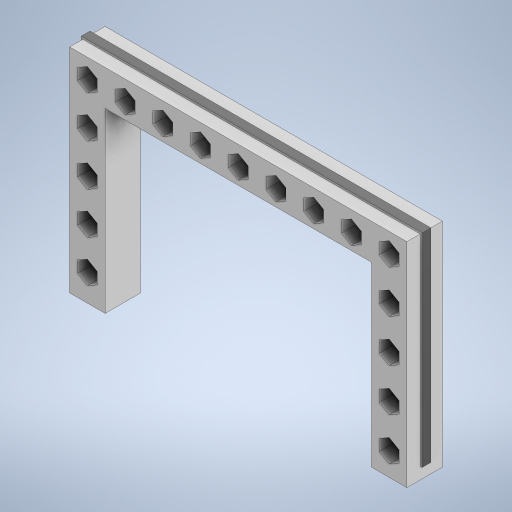
# Autodesk Inventor part: estructura
Saved by Autodesk Inventor 2023 (Build 270158000, 158)
## iProperties
Created: 2022-04-04
Part Number: estructura
Material: Genérico
Document SubType Name: Modeling
Designer: isaac
Density: 1 g/cm^3
Appearance: Valor por defecto
Author: isaac
Autodesk Inventor part; units mm, degrees
ref_plane "YZ Plane" through (0, 0, 0) normal (1, 0, 0) x (0, 1, 0)
ref_plane "XZ Plane" through (0, 0, 0) normal (0, 1, 0) x (-1, 0, 0)
ref_plane "XY Plane" through (0, 0, 0) normal (0, 0, 1) x (1, 0, 0)
sketch "Boceto1" plane through (0, 0, 0) normal (0, 0, 1) x (1, 0, 0)
  line L0 (-1500, 0) -> (-1900, 0)
  line L1 (-1900, 0) -> (-1900, 2000)
  line L2 (-1500, 2000) -> (1500, 2000)
  line L3 (1500, 2000) -> (1500, 0)
  line L4 (1500, 0) -> (1900, 0)
  line L5 (1900, 0) -> (1900, 2400)
  line L6 (1900, 2400) -> (-1900, 2400)
  line L7 (-1900, 2400) -> (-1900, 2000)
  line L8 (-1500, 0) -> (-1500, 2000)
  point P0 (0, 0)
  point P1 (0, 2400)
  dimension "d0" = 400
  dimension "d2" = 3000
  dimension "d3" = 400
  dimension "d4" = 2400
  dimension "d5" = 400
  dimension "d6" = 2400
  constraints: 18 end point, 6 perpendicular, 1 horizontal, 1 horizontal alignment, 1 midpoint, 1 point on line, 1 vertical, 1 vertical alignment
  measures "d0" distance of L0.start L0.end
  measures "d2" distance of L2.start L2.end
  measures "d3" distance of L3.end L4.end
  measures "d4" distance of L4.end L5.end
  measures "d5" distance between parallel lines of L2 L6
  measures "d6" distance between parallel lines of L0 L6
extrude "Extrusión1" add sketch "Boceto1" along normal mid plane 400
sketch "Boceto2" plane through (0, 0, 200) normal (0, 0, 1) x (1, 0, 0)
  line L0 (-1700, 429.3142) -> (-1588.0106, 364.6571)
  line L1 (-1588.0106, 364.6571) -> (-1588.0106, 235.3429)
  line L2 (-1588.0106, 235.3429) -> (-1700, 170.6858)
  line L3 (-1700, 170.6858) -> (-1811.9894, 235.3429)
  line L4 (-1811.9894, 235.3429) -> (-1811.9894, 364.6571)
  line L5 (-1811.9894, 364.6571) -> (-1700, 429.3142)
  line L6 (1500, 2000) -> (1500, 0) construction
  line L7 (1500, 0) -> (1900, 0) construction
  line L8 (1900, 0) -> (1900, 2400) construction
  line L9 (1900, 2400) -> (-1900, 2400) construction
  line L10 (-1900, 2400) -> (-1900, 0) construction
  line L11 (-1900, 0) -> (-1500, 0) construction
  line L12 (-1500, 0) -> (-1500, 2000) construction
  line L13 (-1500, 2000) -> (1500, 2000) construction
  line L14 (-1588.0106, 834.6571) -> (-1588.0106, 705.3429)
  line L15 (-1700, 899.3142) -> (-1588.0106, 834.6571)
  line L16 (-1588.0106, 705.3429) -> (-1700, 640.6858)
  line L17 (-1811.9894, 834.6571) -> (-1700, 899.3142)
  line L18 (-1811.9894, 705.3429) -> (-1811.9894, 834.6571)
  line L19 (-1700, 640.6858) -> (-1811.9894, 705.3429)
  line L20 (-1588.0106, 1304.6571) -> (-1588.0106, 1175.3429)
  line L21 (-1700, 1369.3142) -> (-1588.0106, 1304.6571)
  line L22 (-1588.0106, 1175.3429) -> (-1700, 1110.6858)
  line L23 (-1811.9894, 1304.6571) -> (-1700, 1369.3142)
  line L24 (-1811.9894, 1175.3429) -> (-1811.9894, 1304.6571)
  line L25 (-1700, 1110.6858) -> (-1811.9894, 1175.3429)
  line L26 (-1588.0106, 1774.6571) -> (-1588.0106, 1645.3429)
  line L27 (-1700, 1839.3142) -> (-1588.0106, 1774.6571)
  line L28 (-1588.0106, 1645.3429) -> (-1700, 1580.6858)
  line L29 (-1811.9894, 1774.6571) -> (-1700, 1839.3142)
  line L30 (-1811.9894, 1645.3429) -> (-1811.9894, 1774.6571)
  line L31 (-1700, 1580.6858) -> (-1811.9894, 1645.3429)
  line L32 (-1588.0106, 2244.6571) -> (-1588.0106, 2115.3429)
  line L33 (-1700, 2309.3142) -> (-1588.0106, 2244.6571)
  line L34 (-1588.0106, 2115.3429) -> (-1700, 2050.6858)
  line L35 (-1811.9894, 2244.6571) -> (-1700, 2309.3142)
  line L36 (-1811.9894, 2115.3429) -> (-1811.9894, 2244.6571)
  line L37 (-1700, 2050.6858) -> (-1811.9894, 2115.3429)
  line L38 (-1275, 2050.6858) -> (-1386.9894, 2115.3429)
  line L39 (-1163.0106, 2244.6571) -> (-1163.0106, 2115.3429)
  line L40 (-1386.9894, 2115.3429) -> (-1386.9894, 2244.6571)
  line L41 (-1386.9894, 2244.6571) -> (-1275, 2309.3142)
  line L42 (-1275, 2309.3142) -> (-1163.0106, 2244.6571)
  line L43 (-1163.0106, 2115.3429) -> (-1275, 2050.6858)
  line L44 (-850, 2050.6858) -> (-961.9894, 2115.3429)
  line L45 (-738.0106, 2244.6571) -> (-738.0106, 2115.3429)
  line L46 (-961.9894, 2115.3429) -> (-961.9894, 2244.6571)
  line L47 (-961.9894, 2244.6571) -> (-850, 2309.3142)
  line L48 (-850, 2309.3142) -> (-738.0106, 2244.6571)
  line L49 (-738.0106, 2115.3429) -> (-850, 2050.6858)
  line L50 (-425, 2050.6858) -> (-536.9894, 2115.3429)
  line L51 (-313.0106, 2244.6571) -> (-313.0106, 2115.3429)
  line L52 (-536.9894, 2115.3429) -> (-536.9894, 2244.6571)
  line L53 (-536.9894, 2244.6571) -> (-425, 2309.3142)
  line L54 (-425, 2309.3142) -> (-313.0106, 2244.6571)
  line L55 (-313.0106, 2115.3429) -> (-425, 2050.6858)
  line L56 (0, 2050.6858) -> (-111.9894, 2115.3429)
  line L57 (111.9894, 2244.6571) -> (111.9894, 2115.3429)
  line L58 (-111.9894, 2115.3429) -> (-111.9894, 2244.6571)
  line L59 (-111.9894, 2244.6571) -> (0, 2309.3142)
  line L60 (0, 2309.3142) -> (111.9894, 2244.6571)
  line L61 (111.9894, 2115.3429) -> (0, 2050.6858)
  line L62 (425, 2050.6858) -> (313.0106, 2115.3429)
  line L63 (536.9894, 2244.6571) -> (536.9894, 2115.3429)
  line L64 (313.0106, 2115.3429) -> (313.0106, 2244.6571)
  line L65 (313.0106, 2244.6571) -> (425, 2309.3142)
  line L66 (425, 2309.3142) -> (536.9894, 2244.6571)
  line L67 (536.9894, 2115.3429) -> (425, 2050.6858)
  line L68 (850, 2050.6858) -> (738.0106, 2115.3429)
  line L69 (961.9894, 2244.6571) -> (961.9894, 2115.3429)
  line L70 (738.0106, 2115.3429) -> (738.0106, 2244.6571)
  line L71 (738.0106, 2244.6571) -> (850, 2309.3142)
  line L72 (850, 2309.3142) -> (961.9894, 2244.6571)
  line L73 (961.9894, 2115.3429) -> (850, 2050.6858)
  line L74 (1275, 2050.6858) -> (1163.0106, 2115.3429)
  line L75 (1386.9894, 2244.6571) -> (1386.9894, 2115.3429)
  line L76 (1163.0106, 2115.3429) -> (1163.0106, 2244.6571)
  line L77 (1163.0106, 2244.6571) -> (1275, 2309.3142)
  line L78 (1275, 2309.3142) -> (1386.9894, 2244.6571)
  line L79 (1386.9894, 2115.3429) -> (1275, 2050.6858)
  line L80 (1700, 2050.6858) -> (1588.0106, 2115.3429)
  line L81 (1811.9894, 2244.6571) -> (1811.9894, 2115.3429)
  line L82 (1588.0106, 2115.3429) -> (1588.0106, 2244.6571)
  line L83 (1588.0106, 2244.6571) -> (1700, 2309.3142)
  line L84 (1700, 2309.3142) -> (1811.9894, 2244.6571)
  line L85 (1811.9894, 2115.3429) -> (1700, 2050.6858)
  line L86 (1588.0106, 1635.3429) -> (1588.0106, 1764.6571)
  line L87 (1700, 1570.6858) -> (1588.0106, 1635.3429)
  line L88 (1588.0106, 1764.6571) -> (1700, 1829.3142)
  line L89 (1811.9894, 1635.3429) -> (1700, 1570.6858)
  line L90 (1811.9894, 1764.6571) -> (1811.9894, 1635.3429)
  line L91 (1700, 1829.3142) -> (1811.9894, 1764.6571)
  line L92 (1588.0106, 1155.3429) -> (1588.0106, 1284.6571)
  line L93 (1700, 1090.6858) -> (1588.0106, 1155.3429)
  line L94 (1588.0106, 1284.6571) -> (1700, 1349.3142)
  line L95 (1811.9894, 1155.3429) -> (1700, 1090.6858)
  line L96 (1811.9894, 1284.6571) -> (1811.9894, 1155.3429)
  line L97 (1700, 1349.3142) -> (1811.9894, 1284.6571)
  line L98 (1588.0106, 675.3429) -> (1588.0106, 804.6571)
  line L99 (1700, 610.6858) -> (1588.0106, 675.3429)
  line L100 (1588.0106, 804.6571) -> (1700, 869.3142)
  line L101 (1811.9894, 675.3429) -> (1700, 610.6858)
  line L102 (1811.9894, 804.6571) -> (1811.9894, 675.3429)
  line L103 (1700, 869.3142) -> (1811.9894, 804.6571)
  line L104 (1588.0106, 195.3429) -> (1588.0106, 324.6571)
  line L105 (1700, 130.6858) -> (1588.0106, 195.3429)
  line L106 (1588.0106, 324.6571) -> (1700, 389.3142)
  line L107 (1811.9894, 195.3429) -> (1700, 130.6858)
  line L108 (1811.9894, 324.6571) -> (1811.9894, 195.3429)
  line L109 (1700, 389.3142) -> (1811.9894, 324.6571)
  point P0 (0, 0)
  point P1 (-1700, 300)
  point P2 (-1700, 770)
  point P3 (-1700, 1240)
  point P4 (-1700, 1710)
  point P5 (-1700, 2180)
  point P6 (-1275, 2180)
  point P7 (-850, 2180)
  point P8 (-425, 2180)
  point P9 (0, 2180)
  point P10 (425, 2180)
  point P11 (850, 2180)
  point P12 (1275, 2180)
  point P13 (1700, 2180)
  point P14 (1700, 1700)
  point P15 (1700, 1220)
  point P16 (1700, 740)
  point P17 (1700, 260)
  dimension "d9" = 300
  dimension "d10" = 200
  dimension "d11" = 64.6571
  dimension "d14" = 470
  dimension "d21" = 425
  dimension "d28" = 480
  constraints: 204 end point, 2 vertical, 1 horizontal, 1 horizontal alignment, 1 vertical alignment, 221 other
  measures "d9" distance from line of L11 point (-1700, 300)
  measures "d10" distance from line of L10 point (-1700, 300)
  measures "d11" vertical distance of L1.end L2.end
  measures "d14" distance of L0.end L14.start
  measures "d21" distance of L34.end L38.start
  measures "d28" distance of L80.end L86.start
extrude "Extrusión2" cut sketch "Boceto2" against normal blind 400
sketch "Boceto5" plane through (1900, 0, 200) normal (1, 0, 0) x (0, 0, -1)
  line L0 (400, 2400) -> (0, 2400) construction
  line L1 (0, 0) -> (0, 2400) construction
  line L2 (400, 0) -> (0, 0) construction
  line L3 (400, 2400) -> (400, 0) construction
  line L4 (0, 130.6858) -> (400, 130.6858) construction
  line L5 (400, 2400) -> (0, 2400) construction
  line L6 (150, 130.6858) -> (250, 130.6858)
  line L7 (250, 130.6858) -> (250, 2400)
  line L8 (250, 2400) -> (150, 2400)
  line L9 (150, 2400) -> (150, 130.6858)
  point P0 (200, 0)
  dimension "d42" = 100
  dimension "d43" = 150
  constraints: 8 end point, 2 parallel, 2 point on line, 1 horizontal, 1 perpendicular
  measures "d42" distance between parallel lines of L7 L9
  measures "d43" distance between parallel lines of L1 L9
extrude "Extrusión3" add sketch "Boceto5" along normal blind 20
sketch "Boceto6" plane through (-1900, 2400, 200) normal (0, 1, 0) x (1, 0, 0)
  line L0 (0, 400) -> (0, 0) construction
  line L1 (3800, 0) -> (0, 0) construction
  line L2 (3800, 150) -> (3800, 0) construction
  line L3 (3800, 150) -> (3820, 150) construction
  line L4 (3820, 250) -> (3820, 150) construction
  line L5 (3800, 250) -> (3820, 250) construction
  line L6 (3800, 400) -> (3800, 250) construction
  line L7 (0, 400) -> (3800, 400) construction
  line L8 (3820, 250) -> (-20, 250)
  line L9 (-20, 250) -> (-20, 150)
  line L10 (-20, 150) -> (3820, 150)
  line L11 (3820, 150) -> (3820, 250)
  point P0 (1900, 200)
  dimension "d46" = 3840
  dimension "d47" = 100
  constraints: 8 end point, 2 parallel, 1 horizontal, 1 perpendicular
  measures "d46" distance between parallel lines of L4 L9
  measures "d47" distance between parallel lines of L10 L8
extrude "Extrusión4" add sketch "Boceto6" along normal blind 20
sketch "Boceto7" plane through (-1900, 0, 200) normal (-1, 0, 0) x (0, 0, 1)
  line L0 (-400, 0) -> (0, 0) construction
  line L1 (0, 2400) -> (0, 0) construction
  line L2 (-150, 2400) -> (0, 2400) construction
  line L3 (-250, 2400) -> (-150, 2400) construction
  line L4 (-400, 2400) -> (-250, 2400) construction
  line L5 (-400, 0) -> (-400, 2400) construction
  line L6 (-250, 2400) -> (-150, 2400) construction
  line L7 (-150, 2400) -> (-150, 2420) construction
  line L8 (-250, 2420) -> (-150, 2420) construction
  line L9 (-250, 2400) -> (-250, 2420) construction
  line L10 (-150, 2400) -> (-250, 2400)
  line L11 (-250, 2400) -> (-250, 0)
  line L12 (-250, 0) -> (-150, 0)
  line L13 (-150, 0) -> (-150, 2400)
  point P0 (-200, 0)
  dimension "d50" = 100
  constraints: 8 end point, 2 parallel, 1 horizontal, 1 perpendicular, 1 point on line
  measures "d50" distance between parallel lines of L11 L13
extrude "Extrusión5" add sketch "Boceto7" along normal blind 20
